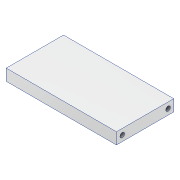
# Autodesk Inventor part: Soporte para culata carcasa
Saved by Autodesk Inventor 2020 (Build 240168000, 168)
## iProperties
Created: 2020-08-06
Part Number: Soporte para culata carcasa
Material: Aluminio 6061
Document SubType Name: Modeling
Designer: Pipi
Density: 2.7 g/cm^3
Appearance: Aluminio - Plano
Author: Pipi
Autodesk Inventor part; units mm, degrees
ref_plane "YZ Plane" through (0, 0, 0) normal (1, 0, 0) x (0, 1, 0)
ref_plane "XZ Plane" through (0, 0, 0) normal (0, 1, 0) x (-1, 0, 0)
ref_plane "XY Plane" through (0, 0, 0) normal (0, 0, 1) x (1, 0, 0)
sketch "Boceto1" plane through (0, 0, 0) normal (0, 1, 0) x (-1, 0, 0)
  line L0 (9.3742, 70.1532) -> (-86.8258, 70.1532)
  line L1 (-86.8258, 70.1532) -> (-86.8258, 20.1532)
  line L2 (-86.8258, 20.1532) -> (9.3742, 20.1532)
  line L3 (9.3742, 20.1532) -> (9.3742, 70.1532)
  dimension "d0" = 96.2
  dimension "d1" = 50
  constraints: 8 end point, 2 parallel, 1 horizontal, 1 perpendicular
  measures "d0" distance of L2.end L1.end
  measures "d1" distance between parallel lines of L2 L0
extrude "Extrusión1" add sketch "Boceto1" along normal blind 10
sketch "Boceto2" plane through (86.8258, 0, 70.1532) normal (1, 0, 0) x (0, 0, -1)
  line L0 (0, 0) -> (0, 10) projected
  line L1 (50, 0) -> (50, 10) projected
  circle A0 centre (5, 5) radius 2
  circle A1 centre (45, 5) radius 2
  point P0 (70.1532, 0)
  dimension "d4" = 4
  dimension "d5" = 5
  dimension "d6" = 4
  dimension "d7" = 5
  constraints: 2 centre point
  measures "d4" diameter of A0
  measures "d5" distance from line of L0 A0.centre
  measures "d6" diameter of A1
  measures "d7" distance from line of L1 A1.centre
sketch "Boceto3" plane through (-9.3742, 0, 20.1532) normal (-1, 0, 0) x (0, 0, 1)
  circle A0 centre (5, 5) radius 2
  line L0 (0, 10) -> (50, 10) projected
  line L1 (0, 0) -> (0, 10) projected
  circle A1 centre (45, 5) radius 2
  line L2 (50, 0) -> (50, 10) projected
  dimension "d8" = 4
  dimension "d9" = 5
  dimension "d10" = 5
  dimension "d11" = 4
  dimension "d12" = 5
  dimension "d13" = 5
  constraints: 2 centre point
  measures "d8" diameter of A0
  measures "d9" distance from line of L0 A0.centre
  measures "d10" distance from line of L1 A0.centre
  measures "d11" diameter of A1
  measures "d12" distance from line of L2 A1.centre
  measures "d13" distance from line of L0 A1.centre
hole "Agujero1" at (-9.3742, 5, 25.1532) at (-9.3742, 5, 65.1532) direction (1, 0, 0) diameter 4 depth 10 tip angle 118
hole "Agujero2" at (86.8258, 5, 65.1532) at (86.8258, 5, 25.1532) direction (-1, 0, 0) diameter 4 depth 10 tip angle 118
thread "Rosca1" size "M4x0.7" class "6H" standard "ISO Metric profile" length 7.5
thread "Rosca2" size "M4x0.7" class "6H" standard "ISO Metric profile" length 7.5
thread "Rosca3" size "M4x0.7" class "6H" standard "ISO Metric profile" length 7.5
thread "Rosca4" size "M4x0.7" class "6H" standard "ISO Metric profile" length 7.5
